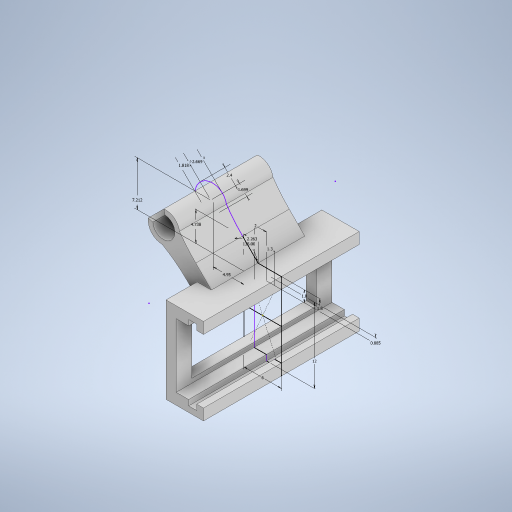
# Autodesk Inventor part: led-mount
Saved by Autodesk Inventor 2023 (Build 270158000, 158)
## iProperties
Created: 2023-02-22
Part Number: led-mount
Material: Generisch
Document SubType Name: Modeling
Designer: tommi
Density: 1 g/cm^3
Appearance: Vorgabe
Author: tommi
## iProperties of the stored document led-mount_3D-Druck.ipt
Created: 2023-02-23
Part Number: led-mount_3D-Druck
Material: Generisch
Document SubType Name: Modeling
Designer: tommi
Density: 1 g/cm^3
Appearance: Vorgabe
Author: tommi
Autodesk Inventor part; units mm, degrees
ref_plane "YZ Plane" through (0, 0, 0) normal (1, 0, 0) x (0, 1, 0)
ref_plane "XZ Plane" through (0, 0, 0) normal (0, 1, 0) x (-1, 0, 0)
ref_plane "XY Plane" through (0, 0, 0) normal (0, 0, 1) x (1, 0, 0)
sketch "Skizze1" plane through (0, 0, 0) normal (0, 0, 1) x (1, 0, 0)
  line L0 (-0.7373, 6.915) -> (3, 6.915)
  line L1 (3, 6.915) -> (3, -6.915)
  line L2 (3, -6.915) -> (-3, -6.915)
  line L3 (-3, -6.915) -> (-3, 4.6523)
  line L4 (-3, 6.915) -> (3, -6.915) construction
  line L5 (3, 6.915) -> (-3, -6.915) construction
  line L6 (-3, 0) -> (3, 0)
  line L7 (1.925, 6) -> (1.925, 5.115)
  line L8 (0.625, 6) -> (0.625, 5.115)
  line L9 (-1.375, 5.115) -> (-1.375, 0)
  line L10 (0.625, 6) -> (1.925, 6)
  line L11 (-1.375, 5.115) -> (0.625, 5.115)
  line L12 (1.925, 5.115) -> (3, 5.115)
  line L13 (-3, 0) -> (3, 0)
  line L14 (0.625, -6) -> (0.625, -5.115)
  line L15 (-1.375, -5.115) -> (-1.375, 0)
  line L16 (0.625, -6) -> (1.925, -6)
  line L17 (-1.375, -5.115) -> (0.625, -5.115)
  line L18 (1.925, -5.115) -> (3, -5.115)
  line L19 (1.925, -5.115) -> (1.925, -6)
  line L20 (-3, 6.915) -> (2.008, 6.915) construction
  line L21 (-3, 6.915) -> (4, 6.915) construction
  line L22 (-3, 6.915) -> (-7.9497, 11.8647)
  line L23 (-3, 6.915) -> (4, 6.915) construction
  line L24 (-0.7373, 6.915) -> (-3.3906, 9.5683)
  line L25 (-4.5789, 6.2311) -> (-3, 4.6523)
  ellipse E0 centre (-8.3445, 11.8647) end of major axis (-7.059, 13.1503) minor radius 1.6987
  ellipse E1 centre (-8.3445, 11.8647) end of major axis (-6.4572, 13.7521) minor radius 2.3999
  arc A0 (-4.5682, 6.2204) -> (-8.6297, 9.3267) centre (-18.2185, -7.4192) ccw
  arc A1 (-5.8407, 12.5429) -> (-3.2355, 9.4133) centre (11.6468, 24.4506) ccw
  line L26 (-8.1548, 13.6227) -> (-10.1025, 11.6751)
  line L27 (-8.1548, 13.6227) -> (-8.3445, 14.3886)
  line L28 (-8.3445, 14.3886) -> (-10.8684, 11.8647)
  line L29 (-10.1025, 11.6751) -> (-10.8684, 11.8647)
  line L30 (-3, 4.6523) -> (-3, 6.915)
  line L31 (-3, 6.915) -> (-0.7373, 6.915)
  point P0 (0, 0)
  point P1 (1.925, 5.5575)
  point P2 (-8.5245, 12.4395)
  point P3 (3, -5.115)
  point P4 (1.275, -6)
  point P5 (1.275, 6)
  point P6 (2.4625, 5.115)
  point P7 (-5.4749, 9.3899)
  dimension "d34" = 1.6987
  dimension "d35" = 1.818
  dimension "d36" = 2.6691
  dimension "d37" = 2.4
  dimension "d0" = 6
  dimension "d19" = 1.3
  dimension "d20" = 2
  dimension "d26" = 1.8
  dimension "d27" = 1.8
  dimension "d30" = 135
  dimension "d40" = 12
  dimension "d41" = 0.885
  dimension "d44" = 7.2125
  dimension "d45" = 4.9497
  dimension "d46" = 4.7376
  dimension "d47" = 2.2627
  constraints: 64 end point, 8 midpoint, 7 point on line, 6 perpendicular, 6 point on circle, 6 symmetric about line, 5 parallel, 4 horizontal, 3 vertical, 2 centre point, 1 coincident, 1 collinear, 1 equal length, 13 other
  measures "d0" distance of L1.end L2.end
  measures "d19" distance between parallel lines of L7 L8
  measures "d20" distance between parallel lines of L9 L8
  measures "d26" distance between parallel lines of L0 L12
  measures "d27" distance between parallel lines of L20 L11
  measures "d30" angle of L23 L22
  measures "d40" distance of point (1.275, -6) point (1.275, 6)
  measures "d41" distance from line of L10 point (2.462, 5.115)
  measures "d44" vertical distance of point (-8.345, 11.865) L3.end
  measures "d45" distance from line of L3 L22.end
  measures "d46" vertical distance of L3.end point (-5.475, 9.39)
  measures "d47" distance of L4.start L0.start
extrude "Extrusion1" add sketch "Skizze1" along normal mid plane 15 contours L31 L22 E1 A1 L24 | L30 L25 A0 E1 L22 | E1 L29 E0 L22 | L22 E0 L27 E1
extrude "Extrusion2" add sketch "Skizze1" along normal mid plane 25 contours L0 L1 L12 L7 L10 L8 L11 L9 L6 L3 L30 L31 | L6 L15 L17 L14 L16 L19 L18 L1 L2 L3
sketch "Skizze2" plane through (-3, -6.915, -12.5) normal (-1, 0, 0) x (0, 0, 1)
  line L0 (2.5, 11.33) -> (22.5, 11.33)
  line L1 (22.5, 11.33) -> (22.5, 2.5)
  line L2 (22.5, 2.5) -> (2.5, 2.5)
  line L3 (2.5, 2.5) -> (2.5, 11.33)
  line L4 (2.5, 11.33) -> (22.5, 2.5) construction
  line L5 (22.5, 11.33) -> (2.5, 2.5) construction
  line L6 (0, 0) -> (0, 13.83) projected
  line L7 (0, 0) -> (25, 0) projected
  point P0 (12.5, 6.915)
  point P1 (12.5, 2.5)
  dimension "d50" = 2.5
  dimension "d51" = 2.5
  constraints: 12 end point, 3 midpoint, 2 parallel, 1 horizontal, 1 perpendicular
  measures "d50" distance between parallel lines of L6 L3
  measures "d51" distance from line of L7 point (12.5, 2.5)
extrude "Extrusion3" cut sketch "Skizze2" against normal up to surface (1.625 mm away)
